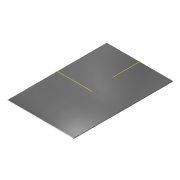
# Autodesk Inventor part: 00_Astromedia_FronSurfaceMirror_120x80mmx1mm
Saved by Autodesk Inventor 2022.5 (Build 265521000, 521)
## iProperties
Created: 2022-07-29
Part Number: 00_Astromedia_FronSurfaceMirror_120x80mmx1mm
Material: Generisch
Document SubType Name: Modeling
Designer: UC2
Density: 1 g/cm^3
Appearance: Chrom - poliert
Catalog Web Link: https://astromedia.de/Vorderflaechen-Glasspiegel-40x30mm
Vendor: Astromedia
Mass: 1.2 g
Surface Area: 25.4 cm^2
Volume: 1.2 cm^3
Author: UC2
Autodesk Inventor part; units mm, degrees
ref_plane "YZ Plane" through (0, 0, 0) normal (1, 0, 0) x (0, 1, 0)
ref_plane "XZ Plane" through (0, 0, 0) normal (0, 1, 0) x (-1, 0, 0)
ref_plane "XY Plane" through (0, 0, 0) normal (0, 0, 1) x (1, 0, 0)
sketch "Skizze1" plane through (0, 0, 0) normal (0, 1, 0) x (-1, 0, 0)
  line L0 (-40, -60) -> (40, -60)
  line L1 (40, -60) -> (40, 60)
  line L2 (40, 60) -> (-40, 60)
  line L3 (-40, 60) -> (-40, -60)
  line L4 (-40, -60) -> (40, 60) construction
  line L5 (40, -60) -> (-40, 60) construction
  point P0 (0, 0)
  dimension "d0" = 80
  dimension "d1" = 120
  constraints: 12 end point, 2 midpoint, 2 parallel, 1 horizontal, 1 perpendicular
  measures "d0" distance of L2.end L1.end
  measures "d1" distance of L1.end L0.end
extrude "Extrusion1" add sketch "Skizze1" along normal blind 1
ref_plane "Arbeitsebene1" through (-40, 0, 0) normal (0, 0, 1) x (1, 0, 0)
ref_plane "Arbeitsebene2" through (0, 0, -60) normal (-1, 0, 0) x (0, 0, 1)
